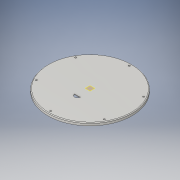
# Autodesk Inventor part: Turntable Cap
Saved by Autodesk Inventor 2016 (Build 200138000, 138)
## iProperties
Created: 2016-04-25
Part Number: Turntable Cap
Material: PVC-Piping
Document SubType Name: Modeling
Designer: rubenjm
Density: 1.4 g/cm^3
Appearance: Smooth - White
Author: rubenjm
Autodesk Inventor part; units mm, degrees
ref_plane "YZ Plane" through (0, 0, 0) normal (1, 0, 0) x (0, 1, 0)
ref_plane "XZ Plane" through (0, 0, 0) normal (0, 1, 0) x (-1, 0, 0)
ref_plane "XY Plane" through (0, 0, 0) normal (0, 0, 1) x (1, 0, 0)
sketch "Sketch1" plane through (0, 0, 0) normal (0, 1, 0) x (-1, 0, 0)
  circle A0 centre (0, 0) radius 190.5
  dimension "d1" = 381
  constraints: 1 centre point
  measures "d1" diameter of A0
ref_plane "Work Plane1" through (0, 12.7, 0) normal (0, 1, 0) x (1, 0, 0)
sketch "Sketch2" plane through (0, 12.7, 0) normal (0, 1, 0) x (1, 0, 0)
  line L0 (0, 0) -> (0, -177.8) construction
  line L1 (0, 0) -> (177.8, 0) construction
  circle A0 centre (0, -177.8) radius 3.81
  circle A1 centre (153.9793, -88.9) radius 3.81
  circle A2 centre (153.9793, 88.9) radius 3.81
  circle A3 centre (0, 177.8) radius 3.81
  circle A4 centre (-153.9793, 88.9) radius 3.81
  circle A5 centre (-153.9793, -88.9) radius 3.81
  dimension "d6" = 177.8
  dimension "d7" = 90
  dimension "d8" = 7.62
  dimension "d9" = 360
  constraints: 6 centre point, 4 end point, 1 coincident, 1 horizontal, 1 perpendicular, 1 vertical, 13 other
  measures "d6" distance of L0.start L0.end
  measures "d7" angle of L0 L1
  measures "d8" diameter of A0
extrude "Extrusion3" add sketch "Sketch1" along normal blind 12.7
extrude "Extrusion4" cut sketch "Sketch2" against normal through all
sketch "Sketch3" plane through (0, 0, 0) normal (0, -1, 0) x (1, 0, 0)
  circle A0 centre (0, 0) radius 162.56
  dimension "d16" = 325.12
  constraints: 1 centre point, 1 coincident
  measures "d16" diameter of A0
extrude "Extrusion5" cut sketch "Sketch3" against normal blind 9.8806
fillet "Fillet1" radius 3.175 1 edges at (190.5, 12.7, 0)
sketch "Sketch4" plane through (0, 12.7, 0) normal (0, 1, 0) x (1, 0, 0)
  arc A0 (-12.6214, -55.7389) -> (12.6214, -55.7389) centre (0, 0) ccw
  arc A1 (-12.6214, -55.7389) -> (12.6214, -55.7389) centre (0, -57.15) ccw
  dimension "d20" = 114.3
  dimension "d21" = 25.4
  constraints: 5 point on circle, 2 centre point, 1 coincident
  measures "d20" diameter of A0
  measures "d21" diameter of A1
extrude "Extrusion6" cut sketch "Sketch4" against normal blind 9.8806
body "Solid1"
